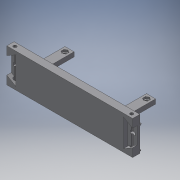
# Autodesk Inventor part: Case_bottom_back
Saved by Autodesk Inventor 2016 SP2 (Build 200236200, 236)
## iProperties
Created: 2018-06-26
Part Number: Case_bottom_back
Material: Generisch
Document SubType Name: Modeling
Designer: Nils
Density: 1 g/cm^3
Appearance: Vorgabe
Author: Nils
Autodesk Inventor part; units mm, degrees
ref_plane "YZ Plane" through (0, 0, 0) normal (1, 0, 0) x (0, 1, 0)
ref_plane "XZ Plane" through (0, 0, 0) normal (0, 1, 0) x (-1, 0, 0)
ref_plane "XY Plane" through (0, 0, 0) normal (0, 0, 1) x (1, 0, 0)
sketch "Skizze1" plane through (0, 0, 0) normal (1, 0, 0) x (0, 1, 0)
  line L0 (-139.6154, -159.9758) -> (-139.6154, -150.6758) projected
  line L1 (-147.6154, -150.6758) -> (-147.6154, -160.0993) projected
  line L2 (-147.6154, -150.6758) -> (-139.6154, -150.6758) projected
  line L3 (-139.6154, -159.9758) -> (-138.1154, -159.9758) projected
  line L4 (-138.1154, -159.9758) -> (-138.1154, -160.4758) projected
  line L5 (-138.1154, -160.4758) -> (-139.6154, -161.9758) projected
  line L6 (-139.6154, -161.9758) -> (-139.6154, -176.9758) projected
  line L7 (-147.6154, -178.5523) -> (-147.6154, -187.9758) projected
  line L8 (-139.6154, -187.9758) -> (-147.6154, -187.9758) projected
  line L9 (-147.6154, -160.0993) -> (-147.6154, -178.5523)
  line L10 (-139.6154, -187.9758) -> (-139.6154, -185.9758)
  line L11 (-139.6154, -185.9758) -> (-138.6154, -185.9758)
  line L12 (-138.6154, -185.9758) -> (-138.6154, -184.9758)
  line L13 (-138.6154, -184.9758) -> (-139.6154, -184.9758)
  line L14 (-139.6154, -184.9758) -> (-139.6154, -176.9758)
  point P0 (0, 0)
  dimension "d19" = 2
  dimension "d20" = 1
  dimension "d21" = 1
  constraints: 12 end point, 3 perpendicular, 2 vertical, 1 collinear, 1 point on line
  measures "d19" distance of L8.start L10.end
  measures "d20" distance of L10.end L11.end
  measures "d21" distance of L11.end L12.end
extrude "Extrusion1" add sketch "Skizze1" along normal blind 69.4
sketch "Skizze2" plane through (0, -147.6154, -187.9758) normal (0, -1, 0) x (1, 0, 0)
  line L0 (0, 27.8765) -> (10, 33.65)
  line L1 (10, 33.65) -> (10, 3.65)
  line L2 (10, 3.65) -> (0, 9.4235)
  line L3 (0, 0) -> (0, 26) projected
  line L4 (0, 27.8765) -> (0, 9.4235)
  line L5 (-0.1, 9.3658) -> (10.1, 3.4768)
  line L6 (10.1, 3.4768) -> (10.1, 33.8232)
  line L7 (10.1, 33.8232) -> (-0.1, 27.9342)
  line L8 (-0.1, 27.9342) -> (-0.1, 9.3658)
  line L9 (10, 33.65) -> (0, 27.8765) projected
  line L10 (10, 33.65) -> (0, 27.8765) projected
  line L11 (10, 3.65) -> (6.4361, 5.7076) projected
  line L12 (0, 9.4235) -> (10, 3.65) projected
  point P0 (0, 187.9758)
  point P1 (-212.8594, 35.25)
  point P2 (-212.8594, 5.25)
  point P3 (-222.8594, 29.4765)
  point P4 (-222.8594, 11.0235)
  dimension "d7" = 0.1
  constraints: 16 end point, 3 collinear, 1 equal length, 1 point on line, 1 vertical, 8 other
  measures "d7" distance between parallel lines of L6 L1
extrude "Extrusion2" cut sketch "Skizze2" against normal blind 5 contours L0 L1 L2 L3 L4 | L8 L7 L6 L5
sketch "Skizze3" plane through (0, -147.6154, -150.6758) normal (0, 0, 1) x (1, 0, 0)
  circle A0 centre (5, 4) radius 1.75 projected
  point P0 (0, 147.6154)
extrude "Extrusion3" cut sketch "Skizze3" against normal blind 35
sketch "Skizze5" plane through (0, -139.6154, -161.9758) normal (0, 1, 0) x (1, 0, 0)
  line L0 (0, 16.692) -> (0, -1.992) projected
  line L1 (7.85, 5.95) -> (2.15, 5.95) projected
  line L2 (2.15, 8.75) -> (7.85, 8.75) projected
  line L3 (2.15, 5.95) -> (2.15, 8.75) projected
  line L4 (7.85, 8.75) -> (7.85, 5.95) projected
  point P0 (0, -161.9758)
  point P1 (-43.8096, 7.15)
  point P2 (0, -11.3)
  constraints: 1 other
extrude "Extrusion4" cut sketch "Skizze5" against normal blind 19.25
sketch "Skizze6" plane through (0, -139.6154, -161.9758) normal (0, 1, 0) x (1, 0, 0)
  line L0 (19.4, 2) -> (29.4, 2)
  line L1 (29.4, 2) -> (29.4, 7)
  line L2 (29.4, 7) -> (19.4, 7)
  line L3 (19.4, 7) -> (19.4, 2)
  line L4 (0, 23) -> (0, 0) projected
  line L5 (0, 0) -> (69.4, 0) projected
  point P0 (0, -161.9758)
  dimension "d22" = 10
  dimension "d23" = 5
  dimension "d24" = 19.4
  dimension "d25" = 2
  constraints: 8 end point, 2 parallel, 1 horizontal, 1 perpendicular
  measures "d22" distance of L2.end L1.end
  measures "d23" distance of L1.end L0.end
  measures "d24" distance between parallel lines of L3 L4
  measures "d25" distance between parallel lines of L5 L0
extrude "Extrusion5" add sketch "Skizze6" along normal blind 36.75
sketch "Skizze7" plane through (19.4, -139.6154, -163.9758) normal (0, 0, 1) x (1, 0, 0)
  circle A0 centre (5, 31.75) radius 1.75
  line L0 (0, 0) -> (0, 36.75) projected
  line L1 (0, 36.75) -> (10, 36.75) projected
  point P0 (-19.4, 139.6154)
  dimension "d28" = 3.5
  dimension "d29" = 5
  dimension "d30" = 5
  constraints: 1 centre point
  measures "d28" diameter of A0
  measures "d29" distance from line of L0 A0.centre
  measures "d30" distance from line of A0.centre L1
extrude "Extrusion6" cut sketch "Skizze7" against normal blind 36.75
mirror "Spiegeln1" about plane through (69.4, -143.3836, -169.4656) normal (1, 0, 0) of "Extrusion6", "Extrusion5", "Extrusion4", "Extrusion3", "Extrusion2", "Extrusion1"
sketch "Skizze8" plane through (19.4, -139.6154, -163.9758) normal (0, 0, 1) x (1, 0, 0)
  circle A0 centre (5, 31.75) radius 1.75 construction
  circle A1 centre (95, 31.75) radius 1.75 construction
  line L0 (7.85, 30.1046) -> (5, 28.4591)
  line L1 (5, 28.4591) -> (2.15, 30.1046)
  line L2 (2.15, 30.1046) -> (2.15, 33.3954)
  line L3 (2.15, 33.3954) -> (5, 35.0409)
  line L4 (5, 35.0409) -> (7.85, 33.3954)
  line L5 (7.85, 33.3954) -> (7.85, 30.1046)
  circle A2 centre (95, 31.75) radius 1.75 projected
  line L6 (92.15, 30.1046) -> (92.15, 33.3954)
  line L7 (92.15, 33.3954) -> (95, 35.0409)
  line L8 (95, 35.0409) -> (97.85, 33.3954)
  line L9 (97.85, 33.3954) -> (97.85, 30.1046)
  line L10 (97.85, 30.1046) -> (95, 28.4591)
  line L11 (95, 28.4591) -> (92.15, 30.1046)
  point P0 (-19.4, 139.6154)
  dimension "d33" = 5.7
  dimension "d34" = 5.7
  constraints: 24 end point, 2 coincident, 2 vertical, 26 other
  measures "d33" distance between parallel lines of L5 L2
  measures "d34" distance between parallel lines of L9 L6
extrude "Extrusion7" cut sketch "Skizze8" against normal blind 2.2
equation "\"d34\" = d33"
